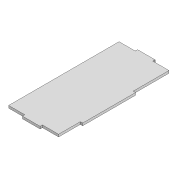
# Autodesk Inventor part: стенка 3
Saved by Autodesk Inventor 2021 (Build 250183000, 183)
## iProperties
Created: 2023-02-14
Part Number: стенка 3
Material: Типовые
Document SubType Name: Modeling
Designer: Tasya
Density: 1 g/cm^3
Appearance: По умолчанию
Author: Tasya
Autodesk Inventor part; units mm, degrees
ref_plane "YZ Plane" through (0, 0, 0) normal (1, 0, 0) x (0, 1, 0)
ref_plane "XZ Plane" through (0, 0, 0) normal (0, 1, 0) x (-1, 0, 0)
ref_plane "XY Plane" through (0, 0, 0) normal (0, 0, 1) x (1, 0, 0)
sketch "Эскиз1" plane through (0, 0, 0) normal (0, 1, 0) x (-1, 0, 0)
  line L0 (97.2595, 134.1284) -> (12.2595, 134.1284)
  line L1 (12.2595, 134.1284) -> (12.2595, -53.8716)
  line L2 (12.2595, -53.8716) -> (97.2595, -53.8716)
  line L3 (97.2595, -53.8716) -> (97.2595, 134.1284)
  line L4 (12.2595, 97.1284) -> (8.2595, 97.1284)
  line L5 (8.2595, 97.1284) -> (8.2595, 7.1284)
  line L6 (8.2595, 7.1284) -> (12.2595, 7.1284)
  line L7 (12.2595, 7.1284) -> (12.2595, 97.1284)
  line L8 (69.7595, 138.1284) -> (39.7595, 138.1284)
  line L9 (39.7595, 138.1284) -> (39.7595, 134.1284)
  line L10 (39.7595, 134.1284) -> (69.7595, 134.1284)
  line L11 (69.7595, 134.1284) -> (69.7595, 138.1284)
  line L12 (69.7595, -53.8716) -> (39.7595, -53.8716)
  line L13 (39.7595, -53.8716) -> (39.7595, -57.8716)
  line L14 (39.7595, -57.8716) -> (69.7595, -57.8716)
  line L15 (69.7595, -57.8716) -> (69.7595, -53.8716)
  line L16 (54.7595, -53.8716) -> (54.7595, -83.5129) construction
  point P0 (-14.3828, -135.2029)
  point P1 (-14.3828, -200.4773)
  point P2 (-14.3828, -47.8079)
  point P3 (-14.3828, 17.4664)
  point P4 (-10.7565, -263.2131)
  point P5 (-3.5038, -263.2131)
  point P6 (-3.5038, 232.8717)
  point P7 (-10.7565, 232.8717)
  point P8 (-3.5038, 79.8397)
  point P9 (-10.7565, 79.8397)
  point P10 (-14.3828, 17.4664)
  point P11 (-14.3828, -47.8079)
  point P12 (-10.7565, -110.1811)
  point P13 (-3.5038, -110.1811)
  point P14 (69.7595, 134.1284)
  point P15 (54.7595, -57.8716)
  point P16 (54.7595, 138.1284)
  dimension "d12" = 4
  dimension "d13" = 90
  dimension "d14" = 85
  dimension "d16" = 37
  dimension "d17" = 30
  dimension "d18" = 4
  dimension "d23" = 61
  constraints: 34 end point, 8 parallel, 5 point on line, 4 horizontal, 4 perpendicular, 3 midpoint, 2 equal length, 1 vertical
  measures "d12" distance of L5.end L6.end
  measures "d13" distance of L4.end L5.end
  measures "d14" distance of L1.end L2.end
  measures "d16" distance between parallel lines of L0 L4
  measures "d17" distance of L8.start L8.end
  measures "d18" distance of L10.end L8.start
  measures "d23" distance between parallel lines of L6 L2
extrude "Выдавливание1" add sketch "Эскиз1" along normal blind 4
